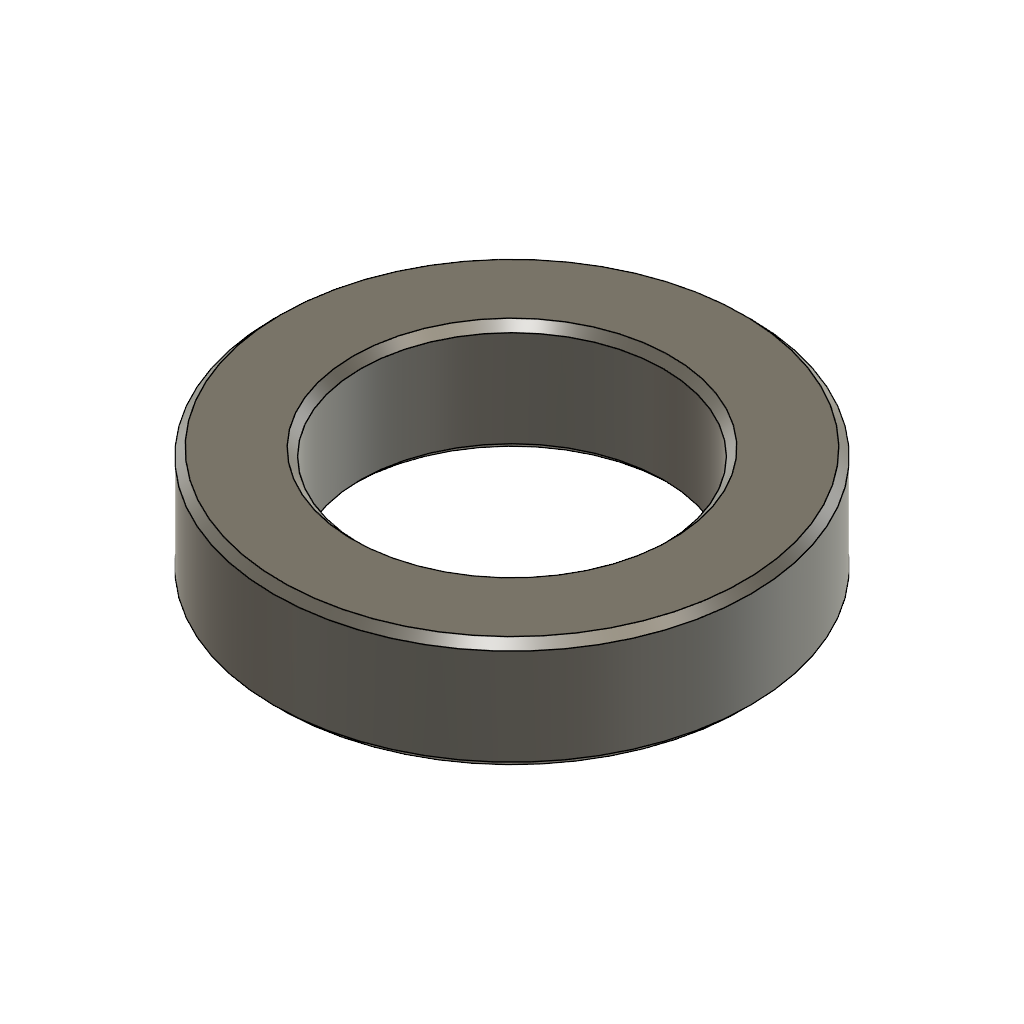
Spacer (Autodesk Fusion 360 design; units mm, degrees)
Autodesk Fusion 360 part; units mm, degrees
sketch "Esboço1" plane through (0, 0, 0) normal (0, 1, 0) x (1, 0, 0)
  circle A0 centre (0, 0) radius 4.1
  circle A1 centre (0, 0) radius 6.45
  dimension "d1" = 8.2
  dimension "d2" = 12.9
  constraint coincident A0.centre A1.centre
  measures "d1" diameter of A0
  measures "d2" diameter of A1
extrude "Extrusão1" add sketch "Esboço1" along normal blind 3
chamfer "Chanfro1" distance 0.2 angle 45 2 edges at (-6.0135, 3, 2.3324) (-6.0135, 0, 2.3324)
chamfer "Chanfro1" distance 0.2 angle 45 2 edges at (-3.8225, 0, -1.4826) (-3.8225, 3, -1.4826)
